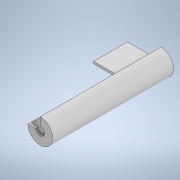
# Autodesk Inventor part: кожух пушки
Saved by Autodesk Inventor 2020.1 (Build 241239000, 239)
## iProperties
Created: 2022-04-02
Part Number: кожух пушки
Material: Типовые
Document SubType Name: Modeling
Designer: User
Density: 1 g/cm^3
Appearance: По умолчанию
Author: User
Autodesk Inventor part; units mm, degrees
ref_plane "YZ Plane" through (0, 0, 0) normal (1, 0, 0) x (0, 1, 0)
ref_plane "XZ Plane" through (0, 0, 0) normal (0, 1, 0) x (-1, 0, 0)
ref_plane "XY Plane" through (0, 0, 0) normal (0, 0, 1) x (1, 0, 0)
sketch "Эскиз1" plane through (0, 0, 0) normal (0, 0, 1) x (1, 0, 0)
  circle A0 centre (0, 0) radius 7.5
  circle A1 centre (0, 0) radius 20
  circle A2 centre (0, 0) radius 22
  line L0 (0, 0) -> (-22, 0)
  line L1 (0, 0) -> (0, 22)
  line L2 (-22, 0) -> (-20, 0)
  line L3 (-20, 0) -> (-20, -4)
  line L4 (-20, -4) -> (-22, -4)
  line L5 (-22, -4) -> (-22, 0)
  point P0 (20, 0)
  point P1 (22, 0)
  point P2 (0, 20)
  point P3 (-20, 0)
  point P4 (-21.6333, -4)
  dimension "d1" = 40
  dimension "d0" = 15
  dimension "d2" = 2
  dimension "d10" = 4
  constraints: 12 end point, 3 coincident, 3 point on circle, 2 centre point, 2 horizontal, 2 parallel, 2 perpendicular, 3 other
  measures "d0" diameter of A0
  measures "d2" distance of A2.start point (20, 0)
  measures "d10" distance of L4.end L0.end
extrude "Выдавливание1" add sketch "Эскиз1" along normal blind 215 contours L1 A2 L4 L3 A1 | L3 L4 A2 L0
sketch "Эскиз2" plane through (0, 0, 215) normal (0, 0, 1) x (1, 0, 0)
  arc A0 (-20, 0) -> (0, 20) centre (0, 0) ccw projected
  arc A1 (-22, 0) -> (0, 22) centre (0, 0) ccw projected
  arc A2 (-22, 0) -> (0, 22) centre (0, 0) ccw projected
  line L0 (0, 22) -> (0, 20) projected
  arc A3 (-20, 0) -> (0, 20) centre (0, 0) ccw projected
  line L1 (-20, 0) -> (-22, 0) projected
  circle A4 centre (0, 0) radius 7.5
  line L2 (0, 7.5) -> (0, 20)
  line L3 (-7.5, 0) -> (-20, 0)
  point P0 (0, 20)
  dimension "d5" = 15
  constraints: 4 end point, 2 point on circle, 1 centre point, 1 coincident, 1 vertical
  measures "d5" diameter of A4
extrude "Выдавливание2" add sketch "Эскиз2" against normal blind 4 contours L3 A4 L2 A0
sketch "Эскиз3" plane through (0, 0, 0) normal (0, 0, -1) x (-1, 0, 0)
  line L0 (20, 0) -> (7.5, 0) projected
  arc A0 (0, 7.5) -> (7.5, 0) centre (0, 0) ccw projected
  line L1 (0, 7.5) -> (0, 20) projected
  arc A1 (0, 20) -> (20, 0) centre (0, 0) ccw projected
extrude "Выдавливание3" add sketch "Эскиз3" against normal blind 4
sketch "Эскиз4" plane through (0, 0, 0) normal (0, 0, -1) x (-1, 0, 0)
  arc A0 (0, 20) -> (20, 0) centre (0, 0) ccw projected
  line L0 (20, 0) -> (60, 0)
  line L1 (60, 0) -> (60, -4)
  line L2 (60, -4) -> (20, -4)
  line L3 (20, -4) -> (20, 0)
  dimension "d11" = 40
  dimension "d12" = 4
  constraints: 8 end point, 2 parallel, 1 horizontal, 1 perpendicular
  measures "d11" distance of L1.end L2.end
  measures "d12" distance of L0.end L1.end
extrude "Выдавливание4" add sketch "Эскиз4" against normal blind 60
